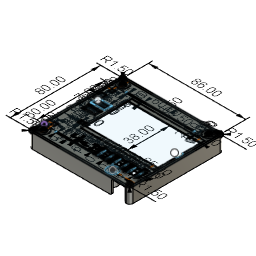
top_cover (Autodesk Fusion 360 design; units mm, degrees)
Autodesk Fusion 360 part; units mm, degrees
sketch "Sketch1" plane through (0, 0, 0) normal (0, 0, 1) x (1, 0, 0)
  line L0 (0, 0) -> (85, 0) construction
  line L1 (85, 0) -> (85, 60) construction
  line L2 (85, 60) -> (0, 60) construction
  line L3 (0, 60) -> (0, 0) construction
  line L4 (19.8, 57.7) -> (83.3, 57.7) construction
  line L5 (83.3, 13.7) -> (19.8, 13.7) construction
  line L6 (19.8, 13.7) -> (19.8, 57.7) construction
  arc A0 (83.3, 32.95) -> (83.3, 38.45) centre (79.5486, 35.7) ccw construction
  line L7 (83.3, 57.7) -> (83.3, 38.45) construction
  line L8 (83.3, 32.95) -> (83.3, 13.7) construction
  line L9 (5.8, 42.2) -> (14.3, 42.2) construction
  line L10 (14.3, 42.2) -> (14.3, 38.8) construction
  line L11 (14.3, 38.8) -> (5.8, 38.8) construction
  line L12 (5.8, 38.8) -> (5.8, 42.2) construction
  line L13 (5.8, 33.8) -> (14.3, 33.8) construction
  line L14 (14.3, 30.4) -> (5.8, 30.4) construction
  line L15 (14.3, 33.8) -> (14.3, 30.4) construction
  line L16 (5.8, 30.4) -> (5.8, 33.8) construction
  line L17 (1.1, 49.8) -> (5.2, 49.8)
  line L18 (5.2, 49.8) -> (5.2, 42.8)
  line L19 (5.2, 42.2) -> (1.1, 42.2)
  line L20 (1.1, 42.2) -> (1.1, 49.8)
  line L21 (71.6, 7.1) -> (82.8, 7.1)
  line L22 (82.8, 7.1) -> (82.8, 0.1)
  line L23 (82.8, 0.1) -> (71.6, 0.1)
  line L24 (71.6, 0.1) -> (71.6, 7.1)
  line L25 (58.4, 0.1) -> (58.4, 7.1)
  line L26 (58.4, 7.1) -> (69.6, 7.1)
  line L27 (69.6, 7.1) -> (69.6, 0.1)
  line L28 (69.6, 0.1) -> (58.4, 0.1)
  line L29 (45.2, 0.1) -> (45.2, 7.1)
  line L30 (56.4, 7.1) -> (56.4, 0.1)
  line L31 (56.4, 0.1) -> (45.2, 0.1)
  line L32 (45.2, 7.1) -> (56.4, 7.1)
  line L33 (39.6, 7.3) -> (44.1, 7.3)
  line L34 (44.1, 7.3) -> (44.1, 1.3)
  line L35 (44.1, 1.3) -> (39.6, 1.3)
  line L36 (39.6, 1.3) -> (39.6, 7.3)
  line L37 (26.5, 4.2) -> (27.5, 4.2) construction
  line L38 (27.5, 4.2) -> (27.5, 2) construction
  line L39 (27.5, 2) -> (26.5, 2) construction
  line L40 (26.5, 2) -> (26.5, 4.2) construction
  line L41 (14.1, 18.8) -> (16.8, 18.8) construction
  line L42 (16.8, 18.8) -> (16.8, 17.3) construction
  line L43 (16.8, 17.3) -> (14.1, 17.3) construction
  line L44 (14.1, 17.3) -> (14.1, 18.8) construction
  line L45 (19.8, 54.7) -> (83.3, 54.7) construction
  line L46 (19.8, 16.7) -> (83.3, 16.7) construction
  line L47 (79.9943, 54.7) -> (79.9943, 57.7) construction
  line L48 (79.9793, 16.7) -> (79.9793, 13.7) construction
  line L49 (1, 70) -> (84, 70)
  line L50 (85.5, 68.5) -> (85.5, -8.5)
  line L51 (84, -10) -> (1, -10)
  line L52 (-0.5, -8.5) -> (-0.5, 68.5)
  line L53 (0, 0) -> (-0.5, 0) construction
  line L54 (85, 0) -> (85.5, 0) construction
  arc A1 (85.5, 68.5) -> (84, 70) centre (84, 68.5) ccw
  arc A2 (1, 70) -> (-0.5, 68.5) centre (1, 68.5) ccw
  line L55 (14.9, 38.2) -> (5.2, 38.2)
  line L56 (5.2, 38.2) -> (5.2, 42.8)
  line L57 (5.2, 42.8) -> (14.9, 42.8)
  line L58 (14.9, 42.8) -> (14.9, 38.2)
  line L59 (14.9, 29.8) -> (5.2, 29.8)
  line L60 (5.2, 29.8) -> (5.2, 34.4)
  line L61 (5.2, 34.4) -> (14.9, 34.4)
  line L62 (14.9, 34.4) -> (14.9, 29.8)
  line L63 (17.1, 17) -> (13.8, 17)
  line L64 (13.8, 17) -> (13.8, 19.1)
  line L65 (13.8, 19.1) -> (17.1, 19.1)
  line L66 (17.1, 19.1) -> (17.1, 17)
  line L67 (26.2, 1.7) -> (26.2, 4.5)
  line L68 (26.2, 4.5) -> (27.8, 4.5)
  line L69 (27.8, 4.5) -> (27.8, 1.7)
  line L70 (27.8, 1.7) -> (26.2, 1.7)
  arc A3 (83.8, 32.791) -> (83.8, 38.609) centre (79.5486, 35.7) ccw
  line L71 (83.8, 58.2) -> (83.8, 38.609)
  line L72 (19.3, 58.2) -> (83.8, 58.2)
  line L73 (19.3, 13.2) -> (19.3, 58.2)
  line L74 (83.8, 13.2) -> (19.3, 13.2)
  line L75 (83.8, 32.791) -> (83.8, 13.2)
  line L76 (83.3, 16.7) -> (83.8, 16.7) construction
  line L77 (19.8, 16.7) -> (19.3, 16.7) construction
  line L78 (19.8, 54.7) -> (19.3, 54.7) construction
  line L79 (83.3, 54.7) -> (83.8, 54.7) construction
  line L80 (19.3, 54.7) -> (83.8, 54.7)
  line L81 (83.8, 16.7) -> (19.3, 16.7)
  line L82 (4.2, 28.8) -> (4.2, 35.4)
  line L83 (4.2, 35.4) -> (15.9, 35.4)
  line L84 (15.9, 35.4) -> (15.9, 28.8)
  line L85 (15.9, 28.8) -> (4.2, 28.8)
  line L86 (15.9, 37.2) -> (4.2, 37.2)
  line L87 (4.2, 37.2) -> (4.2, 42.2)
  line L88 (5.2, 43.8) -> (15.9, 43.8)
  line L89 (15.9, 43.8) -> (15.9, 37.2)
  line L90 (46, 0.1) -> (46, 7.1)
  line L91 (59.2, 0.1) -> (59.2, 7.1)
  line L92 (72.4, 0.1) -> (72.4, 7.1)
  line L93 (82, 7.1) -> (82, 0.1)
  line L94 (68.8, 7.1) -> (68.8, 0.1)
  line L95 (55.6, 7.1) -> (55.6, 0.1)
  line L96 (45.2, 7.9) -> (56.4, 7.9)
  line L97 (58.4, 7.9) -> (69.6, 7.9)
  line L98 (71.6, 7.9) -> (82.8, 7.9)
  line L99 (71.6, 7.9) -> (71.6, 7.1)
  line L100 (82.8, 7.9) -> (82.8, 7.1)
  line L101 (69.6, 7.9) -> (69.6, 7.1)
  line L102 (58.4, 7.9) -> (58.4, 7.1)
  line L103 (56.4, 7.9) -> (56.4, 7.1)
  line L104 (45.2, 7.9) -> (45.2, 7.1)
  line L105 (28.5, 5.2) -> (28.5, 1)
  line L106 (28.5, 1) -> (25.5, 1)
  line L107 (25.5, 1) -> (25.5, 5.2)
  line L108 (25.5, 5.2) -> (28.5, 5.2)
  line L109 (17.8, 16.3) -> (13.1, 16.3)
  line L110 (13.1, 16.3) -> (13.1, 19.8)
  line L111 (13.1, 19.8) -> (17.8, 19.8)
  line L112 (17.8, 19.8) -> (17.8, 16.3)
  arc A4 (-0.5, -8.5) -> (1, -10) centre (1, -8.5) ccw
  arc A5 (84, -10) -> (85.5, -8.5) centre (84, -8.5) ccw
  line L113 (5.0286, 70) -> (5.0286, 60) construction
  line L114 (5, 0) -> (5, -10) construction
  line L115 (3, 57) -> (6, 57)
  line L116 (6, 57) -> (6, 54)
  line L117 (6, 54) -> (3, 54)
  line L118 (3, 54) -> (3, 57)
  line L119 (3.6598, 57) -> (3.6598, 60) construction
  line L120 (3, 56.1331) -> (0, 56.1331) construction
  line L121 (3, 6) -> (6, 6)
  line L122 (6, 6) -> (6, 3)
  line L123 (6, 3) -> (3, 3)
  line L124 (3, 3) -> (3, 6)
  line L125 (3, 4.2552) -> (0, 4.2552) construction
  line L126 (4.6288, 3) -> (4.6288, 0) construction
  circle A6 centre (80.5, 65) radius 4.5
  circle A7 centre (4.5, 65) radius 4.5
  circle A8 centre (4.5, -5) radius 4.5
  circle A9 centre (65.5, -5) radius 4.5
  line L127 (80.5, 70) -> (80.5, 65) construction
  line L128 (80.5, 65) -> (85.5, 65) construction
  line L129 (4.5, -5) -> (4.5, -10) construction
  line L130 (-0.5, -5) -> (4.5, -5) construction
  line L131 (4.5, 65) -> (4.5, 70) construction
  line L132 (4.5, 65) -> (-0.5, 65) construction
  circle A10 centre (80.5, 65) radius 2.45
  circle A11 centre (4.5, 65) radius 2.45
  circle A12 centre (4.5, -5) radius 2.45
  circle A13 centre (65.5, -5) radius 2.45
  line L133 (65.5, -5) -> (85.5, -5) construction
  line L134 (65.5, -5) -> (65.5, -10) construction
  line L135 (11, -0.2) -> (61, -0.2)
  line L136 (61, -0.2) -> (61, -1.2)
  line L137 (61, -1.2) -> (11, -1.2)
  line L138 (11, -1.2) -> (11, -0.2)
  line L139 (11.9151, 61.2) -> (71.9151, 61.2)
  line L140 (71.9151, 61.2) -> (71.9151, 60.2)
  line L141 (71.9151, 60.2) -> (11.9151, 60.2)
  line L142 (11.9151, 60.2) -> (11.9151, 61.2)
  arc A14 (87, 68.5) -> (84, 71.5) centre (84, 68.5) ccw
  line L143 (1, 71.5) -> (84, 71.5)
  arc A15 (1, 71.5) -> (-2, 68.5) centre (1, 68.5) ccw
  line L144 (-2, -8.5) -> (-2, 68.5)
  arc A16 (-2, -8.5) -> (1, -11.5) centre (1, -8.5) ccw
  line L145 (84, -11.5) -> (1, -11.5)
  arc A17 (84, -11.5) -> (87, -8.5) centre (84, -8.5) ccw
  line L146 (87, 68.5) -> (87, -8.5)
  line L147 (80.7, 7.1) -> (80.7, 0.1)
  line L148 (73.7, 7.1) -> (73.7, 0.1)
  line L149 (67.5, 7.1) -> (67.5, 0.1)
  line L150 (60.5, 7.1) -> (60.5, 0.1)
  line L151 (54.3, 7.1) -> (54.3, 0.1)
  line L152 (47.3, 7.1) -> (47.3, 0.1)
  line L153 (82, 5.6203) -> (80.7, 5.6203) construction
  line L154 (73.7, 5.6203) -> (72.4, 5.6203) construction
  line L155 (60.5, 5.995) -> (59.2, 5.995) construction
  line L156 (68.8, 5.995) -> (67.5, 5.995) construction
  line L157 (55.6, 5.995) -> (54.3, 5.995) construction
  line L158 (47.3, 5.995) -> (46, 5.995) construction
  point P0 (-0.5, 70)
  point P1 (85.5, 70)
  point P2 (-0.5, -10)
  dimension "d1" = 85
  dimension "d2" = 60
  dimension "d3" = 63.5
  dimension "d4" = 44
  dimension "d5" = 2.3
  dimension "d6" = 1.7
  dimension "d11" = 8.5
  dimension "d12" = 3.4
  dimension "d13" = 8.5
  dimension "d14" = 3.4
  dimension "d15" = 17.8
  dimension "d16" = 5.8
  dimension "d17" = 5
  dimension "d18" = 5.8
  dimension "d19" = 4.1
  dimension "d20" = 7.6
  dimension "d21" = 1.1
  dimension "d22" = 10.2
  dimension "d23" = 11.2
  dimension "d24" = 7
  dimension "d25" = 2.2
  dimension "d26" = 0.1
  dimension "d27" = 11.2
  dimension "d28" = 7
  dimension "d29" = 11.2
  dimension "d30" = 7
  dimension "d31" = 0.1
  dimension "d32" = 2
  dimension "d33" = 2
  dimension "d34" = 0.1
  dimension "d35" = 4.5
  dimension "d36" = 6
  dimension "d37" = 1.3
  dimension "d38" = 1.1
  dimension "d39" = 1
  dimension "d40" = 2.2
  dimension "d41" = 12.1
  dimension "d42" = 2
  dimension "d43" = 2.7
  dimension "d44" = 1.5
  dimension "d45" = 17.3
  dimension "d46" = 14.1
  dimension "d47" = 38
  dimension "d49" = 86
  dimension "d50" = 80
  dimension "d52" = 1.5
  dimension "d53" = 1.5
  dimension "d55" = -0.6
  dimension "d56" = -0.6
  dimension "d57" = -0.3
  dimension "d58" = -0.3
  dimension "d59" = -0.5
  dimension "d96" = -1.6
  dimension "d105" = 0.8
  dimension "d106" = 0.8
  dimension "d107" = 0.8
  dimension "d108" = 0.8
  dimension "d109" = 0.8
  dimension "d110" = 0.8
  dimension "d111" = -0.8
  dimension "d112" = -0.8
  dimension "d113" = -0.8
  dimension "d122" = -1
  dimension "d123" = -1
  dimension "d140" = 1.5
  dimension "d141" = 1.5
  dimension "d144" = 3
  dimension "d145" = 3
  dimension "d149" = 3
  dimension "d150" = 3
  dimension "d151" = 3
  dimension "d152" = 3
  dimension "d153" = 9
  dimension "d154" = 5
  dimension "d157" = 4.9
  dimension "d158" = 20
  dimension "d159" = 50
  dimension "d160" = 1
  dimension "d161" = 0.2
  dimension "d162" = 60
  dimension "d163" = 1
  dimension "d164" = 0.2
  dimension "d165" = -1.5
  dimension "d178" = 7
  dimension "d179" = 7
  dimension "d180" = 7
  constraint horizontal L0
  constraint vertical L1
  constraint horizontal L2
  constraint vertical L3
  constraint coincident L0.start L3.end
  constraint horizontal L4
  constraint vertical L7
  constraint horizontal L5
  constraint vertical L6
  constraint coincident A0.start L7
  constraint collinear L7 L8
  constraint horizontal L9
  constraint vertical L10
  constraint horizontal L11
  constraint vertical L12
  constraint horizontal L13
  constraint vertical L15
  constraint horizontal L14
  constraint vertical L16
  constraint horizontal L17
  constraint vertical L18
  constraint horizontal L19
  constraint vertical L20
  constraint horizontal L21
  constraint vertical L22
  constraint horizontal L23
  constraint vertical L24
  constraint horizontal L26
  constraint vertical L27
  constraint horizontal L28
  constraint vertical L25
  constraint horizontal L32
  constraint vertical L30
  constraint horizontal L31
  constraint vertical L29
  constraint horizontal L33
  constraint vertical L34
  constraint horizontal L35
  constraint vertical L36
  constraint horizontal L37
  constraint vertical L38
  constraint horizontal L39
  constraint vertical L40
  constraint horizontal L41
  constraint vertical L42
  constraint horizontal L43
  constraint vertical L44
  constraint coincident L6 L45.start
  constraint coincident L7 L45.end
  constraint perpendicular L7 L45
  constraint coincident L6 L46.start
  constraint coincident L8 L46.end
  constraint perpendicular L8 L46
  constraint coincident L45 L47.start
  constraint coincident L4 L47.end
  constraint perpendicular L4 L47
  constraint coincident L46 L48.start
  constraint coincident L5 L48.end
  constraint perpendicular L5 L48
  constraint equal L47 L48
  constraint horizontal L49
  constraint vertical L50
  constraint horizontal L51
  constraint vertical L52
  constraint coincident L52 L53.end
  constraint perpendicular L52 L53
  constraint coincident L50 L54.end
  constraint perpendicular L50 L54
  constraint equal L53 L54
  constraint coincident P1 L49
  constraint coincident P1 L50
  constraint tangent L49 A1
  constraint tangent L50 A1
  constraint coincident P0 L49
  constraint coincident P0 L52
  constraint tangent L49 A2
  constraint tangent L52 A2
  constraint coincident L75 L76.end
  constraint perpendicular L75 L76
  constraint coincident L73 L77.end
  constraint perpendicular L73 L77
  constraint coincident L73 L78.end
  constraint perpendicular L73 L78
  constraint coincident L71 L79.end
  constraint perpendicular L71 L79
  constraint parallel L11 L86
  constraint parallel L12 L87
  constraint parallel L9 L88
  constraint parallel L10 L89
  constraint coincident L18 L88.start
  constraint coincident L19 L87.end
  constraint perpendicular L21 L99
  constraint perpendicular L21 L100
  constraint perpendicular L26 L101
  constraint perpendicular L26 L102
  constraint perpendicular L32 L103
  constraint perpendicular L32 L104
  constraint coincident P2 L51
  constraint coincident P2 L52
  constraint tangent L51 A4
  constraint tangent L52 A4
  constraint tangent L50 A5
  constraint tangent L51 A5
  constraint coincident L49 L113.start
  constraint coincident L2 L113.end
  constraint perpendicular L2 L113
  constraint coincident L0 L114.start
  constraint coincident L51 L114.end
  constraint perpendicular L51 L114
  constraint equal L113 L114
  constraint horizontal L115
  constraint vertical L116
  constraint horizontal L117
  constraint vertical L118
  constraint coincident L115 L119.start
  constraint coincident L2 L119.end
  constraint perpendicular L2 L119
  constraint coincident L118 L120.start
  constraint coincident L3 L120.end
  constraint perpendicular L3 L120
  constraint equal L119 L120
  constraint horizontal L121
  constraint vertical L122
  constraint horizontal L123
  constraint vertical L124
  constraint coincident L124 L125.start
  constraint coincident L3 L125.end
  constraint perpendicular L3 L125
  constraint coincident L123 L126.start
  constraint coincident L0 L126.end
  constraint perpendicular L0 L126
  constraint equal L125 L126
  constraint equal A6 A7
  constraint equal A8 A9
  constraint equal A7 A8
  constraint coincident L49 L127.start
  constraint coincident A6.centre L127.end
  constraint perpendicular L49 L127
  constraint coincident L50 L128.end
  constraint perpendicular L50 L128
  constraint coincident A8.centre L129.start
  constraint coincident L51 L129.end
  constraint perpendicular L51 L129
  constraint coincident L52 L130.start
  constraint perpendicular L129 L130
  constraint coincident A7.centre L131.start
  constraint coincident L49 L131.end
  constraint perpendicular L49 L131
  constraint coincident L52 L132.end
  constraint perpendicular L52 L132
  constraint equal L131 L132
  constraint equal L129 L130
  constraint equal L127 L130
  constraint equal L127 L131
  constraint equal L127 L128
  constraint concentric A6 A10
  constraint concentric A7 A11
  constraint concentric A8 A12
  constraint concentric A9 A13
  constraint equal A10 A13
  constraint equal A12 A13
  constraint equal A10 A11
  constraint coincident A9.centre A13.centre
  constraint coincident L50 L133.end
  constraint perpendicular L50 L133
  constraint coincident L51 L134.end
  constraint perpendicular L51 L134
  constraint equal L127 L134
  constraint horizontal L135
  constraint vertical L136
  constraint horizontal L137
  constraint vertical L138
  constraint horizontal L139
  constraint vertical L140
  constraint horizontal L141
  constraint vertical L142
  constraint coincident L21 L147.start
  constraint coincident L23 L147.end
  constraint perpendicular L23 L147
  constraint coincident L21 L148.start
  constraint coincident L23 L148.end
  constraint perpendicular L23 L148
  constraint coincident L26 L149.start
  constraint coincident L28 L149.end
  constraint perpendicular L28 L149
  constraint coincident L26 L150.start
  constraint coincident L28 L150.end
  constraint perpendicular L26 L150
  constraint coincident L32 L151.start
  constraint coincident L31 L151.end
  constraint perpendicular L31 L151
  constraint coincident L32 L152.start
  constraint coincident L31 L152.end
  constraint perpendicular L31 L152
  constraint coincident L93 L153.start
  constraint coincident L147 L153.end
  constraint perpendicular L147 L153
  constraint coincident L148 L154.start
  constraint coincident L92 L154.end
  constraint perpendicular L92 L154
  constraint coincident L150 L155.start
  constraint coincident L91 L155.end
  constraint perpendicular L91 L155
  constraint coincident L94 L156.start
  constraint coincident L149 L156.end
  constraint perpendicular L149 L156
  constraint coincident L95 L157.start
  constraint coincident L151 L157.end
  constraint perpendicular L151 L157
  constraint coincident L152 L158.start
  constraint coincident L90 L158.end
  constraint perpendicular L90 L158
  constraint equal L153 L154
  constraint equal L155 L156
  constraint equal L157 L158
  measures "d1" distance of L0.start L0.end
  measures "d2" distance of L0.start L2.end
  measures "d3" distance of L4.start L4.end
  measures "d4" distance of L4.start L5.end
  measures "d5" distance of L2 L4
  measures "d6" distance of L1 L7
  measures "d11" distance of L9.start L9.end
  measures "d12" distance of L9.start L11.end
  measures "d13" distance of L13.start L13.end
  measures "d14" distance of L14.end L13.start
  measures "d15" distance of L2 L9
  measures "d16" distance of L3 L12
  measures "d17" distance of L11 L13
  measures "d18" distance of L3 L16
  measures "d19" distance of L17.start L17.end
  measures "d20" distance of L17.start L19.end
  measures "d21" distance of L3 L20
  measures "d22" distance of L2 L17
  measures "d23" distance of L21.start L21.end
  measures "d24" distance of L21.start L23.end
  measures "d25" distance of L1 L22
  measures "d26" distance of L0 L23
  measures "d27" distance of L25.end L26.end
  measures "d28" distance of L25.end L25.start
  measures "d29" distance of L29.end L30.start
  measures "d30" distance of L29.end L29.start
  measures "d31" distance of L0 L28
  measures "d32" distance of L24 L27
  measures "d33" distance of L25 L30
  measures "d34" distance of L0 L31
  measures "d35" distance of L33.start L33.end
  measures "d36" distance of L33.start L35.end
  measures "d37" distance of L0 L35
  measures "d38" distance of L29 L34
  measures "d39" distance of L37.start L37.end
  measures "d40" distance of L37.start L39.end
  measures "d41" distance of L36 L38
  measures "d42" distance of L0 L39
  measures "d43" distance of L41.start L41.end
  measures "d44" distance of L41.start L43.end
  measures "d45" distance of L0 L43
  measures "d46" distance of L3 L44
  measures "d47" distance of L45 L46
  measures "d49" distance of P0 P1
  measures "d50" distance of P0 P2
  measures "d52" radius of A1
  measures "d53" radius of A2
  measures "d140" radius of A4
  measures "d141" radius of A5
  measures "d144" distance of L115.start L115.end
  measures "d145" distance of L115.start L117.end
  measures "d149" distance of L119.start L119.end
  measures "d150" distance of L121.start L121.end
  measures "d151" distance of L121.start L123.end
  measures "d152" distance of L126.start L126.end
  measures "d153" diameter of A6
  measures "d154" distance of L127.start A6.centre
  measures "d157" diameter of A10
  measures "d158" distance of A9.centre L133.end
  measures "d159" distance of L135.start L135.end
  measures "d160" distance of L135.start L137.end
  measures "d161" distance of L0 L135
  measures "d162" distance of L139.start L139.end
  measures "d163" distance of L139.start L141.end
  measures "d164" distance of L2 L141
  measures "d165" distance of A1
  measures "d178" distance of L147 L148
  measures "d179" distance of L149 L150
  measures "d180" distance of L151 L152
extrude "Extrude17" add sketch "Sketch1" against normal blind 13 contours A14 L143 A15 L144 A16 L145 A17 L146 makes body 1
extrude "Extrude16" add sketch "Sketch1" against normal blind 6 separate body contours L135 L136 L137 L138 | L139 L140 L141 L142 makes body 2 at (27.6667, -0.2, -2) makes body 3 at (31.9151, 61.2, -2)
extrude "Extrude15" add sketch "Sketch1" against normal blind 10 separate body contours A6 | A7 | A8 | A9 makes body 4 at (8.9944, -5.2243, -6.6667) makes body 5 at (0.0224, 64.5519, -6.6667) makes body 6 at (66.7188, -0.6682, -6.6667) makes body 7 at (83.6421, 68.2214, -3.3333)
extrude "Extrude14" add sketch "Sketch1" against normal blind 3.4 separate body contours L18 L19 L55 L56 L57 L58 L86 L87 L88 L89 | L21 L98 L99 L100 | L21 L23 L24 L92 | L21 L22 L23 L93 | L25 L26 L28 L91 | L26 L97 L101 L102 | L26 L27 L28 L94 | L29 L31 L32 L90 | L32 L96 L103 L104 | L30 L31 L32 L95 | L82 L83 L84 L85 | L105 L106 L107 L108 | L109 L110 L111 L112 | L115 L116 L117 L118 | L121 L122 L123 L124 makes body 8 at (8.1, 35.4, -1.1333) makes body 9 at (65.8667, 7.9, -2.2667) makes body 10 at (52.6667, 7.9, -2.2667) makes body 11 at (12, 37.2, -1.1333) makes body 12 at (16.2333, 16.3, -1.1333) makes body 13 at (79.0667, 7.9, -2.2667) makes body 14 at (28.5, 2.4, -2.2667) makes body 15 at (4, 57, -1.1333) makes body 16 at (5, 6, -2.2667)
extrude "Extrude13" add sketch "Sketch1" against normal blind 0.6 separate body contours L73 L74 L75 L81 | L71 L72 L73 L80 makes body 17 at (62.3, 55.8667, 0) makes body 18 at (62.3, 15.5333, 0)
extrude "Extrude12" add sketch "Sketch1" against normal blind 1 separate body contours L17 L18 L19 L20 L56 | L21 L23 L92 L148 | L21 L23 L93 L147 | L26 L28 L91 L150 | L26 L28 L94 L149 | L31 L32 L90 L152 | L31 L32 L95 L151 | L33 L34 L35 L36 | L49 L50 L51 L52 A1 A2 A4 A5 | L63 L64 L65 L66 | L67 L68 L69 L70 | A10 | A11 | A12 | A13 makes body 19 at (6.7667, 17.0333, 0) makes body 20 at (16, 17.7, 0) makes body 21 at (26.7333, 2.6333, 0) makes body 22 at (3.1185, 65.513, 0) makes body 23 at (4.2016, -4.2398, 0) makes body 24 at (79.7323, 65.7614, 0) makes body 25 at (64.971, -4.2746, 0)
sketch "Sketch5" plane through (0, -11.5, 0) normal (0, -1, 0) x (1, 0, 0)
  line L0 (84, 0) -> (1, 0)
  line L1 (1, 0) -> (1, -13)
  line L2 (1, -13) -> (84, -13)
  line L3 (84, -13) -> (84, 0)
  line L4 (87, -13, -3) -> (87, -13, 56.0768) construction
  line L5 (85.5, -13, -3) -> (85.5, -13, 45.1939) construction
  line L6 (83, -13) -> (71, -13)
  line L7 (71, -13) -> (71, -1)
  line L8 (71, -1) -> (83, -1)
  line L9 (83, -1) -> (83, -13)
  line L10 (87, 0) -> (87, -13)
  point P0 (87, -13)
  point P1 (85.5, -13)
  dimension "d181" = 12
  dimension "d182" = 1
  dimension "d199" = 4
  constraint coincident P0 L10.end
  constraint horizontal L6
  constraint vertical L7
  constraint horizontal L8
  constraint vertical L9
  constraint coincident L2 L6.start
  measures "d181" distance of L6.start L6.end
  measures "d182" distance of L0 L8
  measures "d199" distance of L9 L10
extrude "Extrude18" cut sketch "Sketch5" against normal blind 1.5 contours L2 L6 L7 L8 L9 bodies 1
fillet "Fillet1" radius 1 1 edges at (83, -10.75, -13) on bodies 1
fillet "Fillet2" radius 1 1 edges at (71, -10.75, -13) on bodies 1
fillet "Fillet3" radius 0.5 1 edges at (83, -10.75, -1) on bodies 1
fillet "Fillet4" radius 0.5 1 edges at (71, -10.75, -1) on bodies 1
fillet "Fillet5" radius 0.1 6 edges at (60.5, 3.6, -1) (67.5, 3.6, -1) (80.7, 3.6, -1) (73.7, 3.6, -1) (47.3, 3.6, -1) (54.3, 3.6, -1) on bodies 19
fillet "Fillet7" radius 0.1 4 edges at (2.2158, -5.886, -10) (2.2158, 64.114, -10) (63.2158, -5.886, -10) (78.2158, 64.114, -10) on bodies 4 5 6 7
